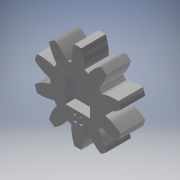
# Autodesk Inventor part: 10_teeth
Saved by Autodesk Inventor 2019 (Build 230136000, 136)
## iProperties
Created: 2020-02-24
Part Number: 10_teeth
Material: Steel
Document SubType Name: Modeling
Designer: Jeff
Categories: <?xml version="1.0" encoding="UTF-16"?> <MemberInstance><Categories><FamilyTemplate><FamilyTemplateParameter ValueType="xs:double" Id="1" ObjectReferenceKey="da_z" ObjectType="kUserParameterObject"/><FamilyTemplateParameter ValueType="xs:double" Id="2" ObjectReferenceKey="da_b" ObjectType="kUserParameterObject"/><FamilyTemplateParameter ValueType="xs:double" Id="3" ObjectReferenceKey="da_beta" ObjectType="kUserParameterObject"/><FamilyTemplateParameter ValueType="xs:double" Id="4" ObjectReferenceKey="da_da" ObjectType="kUserParameterObject"/><FamilyTemplateParameter ValueType="xs:double" Id="5" ObjectReferenceKey="da_aw" ObjectType="kUserParameterObject"/><FamilyTemplateParameter ValueType="xs:string" Id="6" ObjectReferenceKey="EAIAABAAAACIAQAAAAAAAIAAAAAAAAAA" ObjectType="83910656" SubObjectId="SurfaceGeometry"/></FamilyTemplate><ParamToTemplateMap><ParamToTemplate CategoryParameter="//CategoryParameter[@InternalName='046C89C9-8512-4d59-83FE-43B91F4F132A']" TemplateParameter="1"/><ParamToTemplate CategoryParameter="//CategoryParameter[@InternalName='2552DF32-E462-4b46-AEBF-C6C7768E72AC']" TemplateParameter="2"/><ParamToTemplate CategoryParameter="//CategoryParameter[@InternalName='C9EE641D-15FC-4fae-A226-E94C4372FDD7']" TemplateParameter="3"/><ParamToTemplate><ParamToTemplate CategoryParameter="//CategoryParameter[@InternalName='00B6519A-459B-49c7-AD84-2E56D39A5744']" ConstantValue="0.000000"/></ParamToTemplate><ParamToTemplate><ParamToTemplate CategoryParameter="//CategoryParameter[@InternalName='04B31F0E-C7A6-4894-AA32-9629BEFACF47']" ConstantValue="1.000000"/></ParamToTemplate><ParamToTemplate><ParamToTemplate CategoryParameter="//CategoryParameter[@InternalName='43CBEC2E-7847-49e7-A936-2F7889FCB2D9']" ConstantValue="0.250000"/></ParamToTemplate><ParamToTemplate><ParamToTemplate CategoryParameter="//CategoryParameter[@InternalName='B1EFC894-105D-4ebd-86BF-FA20ED196853']" ConstantValue="0.350000"/></ParamToTemplate><ParamToTemplate><ParamToTemplate CategoryParameter="//CategoryParameter[@InternalName='51175063-3D10-4879-93E8-6246FE8B403D']" ConstantValue="2060000000.000000"/></ParamToTemplate><ParamToTemplate><ParamToTemplate CategoryParameter="//CategoryParameter[@InternalName='A3A52E27-4454-46a9-B0BD-C932399B70AF']" ConstantValue="0.300000"/></ParamToTemplate><ParamToTemplate><ParamToTemplate CategoryParameter="//CategoryParameter[@InternalName='91B76062-C214-41d9-B1B9-14D2AB99603D']" ConstantValue="0.300000"/></ParamToTemplate><ParamToTemplate><ParamToTemplate CategoryParameter="//CategoryParameter[@InternalName='374E806E-8B8A-4dda-A9AA-1039D6500AD2']" ConstantValue="3.333333"/></ParamToTemplate><ParamToTemplate><ParamToTemplate CategoryParameter="//CategoryParameter[@InternalName='2D373A89-B862-43d6-8D0B-0CBF12AB9F6C']" ConstantValue="0.349066"/></ParamToTemplate><ParamToTemplate CategoryParameter="//CategoryParameter[@InternalName='37777632-D6A2-4fac-9D53-DB8ACD95C989']" TemplateParameter="4"/><ParamToTemplate CategoryParameter="//CategoryParameter[@InternalName='FD1017F1-B727-4f7e-9707-0F86F1FF9423']" TemplateParameter="5"/><ParamToTemplate><ParamToTemplate CategoryParameter="//CategoryParameter[@InternalName='9E1B4470-B2D3-4ff1-B813-535BB4CDF51A']" ConstantValue="3520000.000000"/></ParamToTemplate><ParamToTemplate><ParamToTemplate CategoryParameter="//CategoryParameter[@InternalName='F8452263-BFF6-458c-9FB1-07C4B99E95CD']" ConstantValue="11400000.000000"/></ParamToTemplate><ParamToTemplate><ParamToTemplate CategoryParameter="//CategoryParameter[@InternalName='3E3BB259-FD49-497f-8171-6EBC954A3479']" ConstantValue="2.000000"/></ParamToTemplate><ParamToTemplate CategoryParameter="//CategoryParameter[@InternalName='27C3BAF2-7550-4e4b-AE2C-0DB134B7D9B7']" TemplateParameter="6"/></ParamToTemplateMap><Category DisplayName="Gear" InternalName="DC85795E-93AB-48d5-8EEE-5A27447B64BD" Mnemonic="Gear"><CategoryParameter DisplayName="z" InternalName="046C89C9-8512-4d59-83FE-43B91F4F132A" Mnemonic="z"/><CategoryParameter DisplayName="b" InternalName="2552DF32-E462-4b46-AEBF-C6C7768E72AC" Mnemonic="b"/><CategoryParameter DisplayName="||b|" InternalName="C9EE641D-15FC-4fae-A226-E94C4372FDD7" Mnemonic="beta"/><CategoryParameter DisplayName="x" InternalName="00B6519A-459B-49c7-AD84-2E56D39A5744" Mnemonic="x"/><CategoryParameter DisplayName="a*" InternalName="04B31F0E-C7A6-4894-AA32-9629BEFACF47" Mnemonic="a"/><CategoryParameter DisplayName="c*" InternalName="43CBEC2E-7847-49e7-A936-2F7889FCB2D9" Mnemonic="c"/><CategoryParameter DisplayName="r|.f|*" InternalName="B1EFC894-105D-4ebd-86BF-FA20ED196853" Mnemonic="rf"/><CategoryParameter DisplayName="E" InternalName="51175063-3D10-4879-93E8-6246FE8B403D" Mnemonic="E"/><CategoryParameter DisplayName="||m|" InternalName="A3A52E27-4454-46a9-B0BD-C932399B70AF" Mnemonic="mi"/><Category DisplayName="SpurGear" InternalName="26C5A22E-A91E-4dfd-A3B3-23CCAFAE1764" Mnemonic="SpurGear"><CategoryParameter DisplayName="m" InternalName="91B76062-C214-41d9-B1B9-14D2AB99603D" Mnemonic="m"/><CategoryParameter DisplayName="P" InternalName="374E806E-8B8A-4dda-A9AA-1039D6500AD2" Mnemonic="PP"/><CategoryParameter DisplayName="||a|" InternalName="2D373A89-B862-43d6-8D0B-0CBF12AB9F6C" Mnemonic="alpha"/><CategoryParameter DisplayName="d|.a|" InternalName="37777632-D6A2-4fac-9D53-DB8ACD95C989" Mnemonic="da"/><CategoryParameter DisplayName="a|.w|" InternalName="FD1017F1-B727-4f7e-9707-0F86F1FF9423" Mnemonic="aw"/><CategoryParameter DisplayName="||s||.Flim|" InternalName="9E1B4470-B2D3-4ff1-B813-535BB4CDF51A" Mnemonic="sFlim"/><CategoryParameter DisplayName="||s||.Hlim|" InternalName="F8452263-BFF6-458c-9FB1-07C4B99E95CD" Mnemonic="sHlim"/><CategoryParameter DisplayName="type" InternalName="3E3BB259-FD49-497f-8171-6EBC954A3479" Mnemonic="type"/><CategoryParameter DisplayName="PitchDiameter" InternalName="27C3BAF2-7550-4e4b-AE2C-0DB134B7D9B7" Mnemonic="IDS_PITCHDIAM"/></Category></Category></Categories></MemberInstance>
Density: 1 g/cm^3
Appearance: Steel
Author: Jeff
Autodesk Inventor part; units mm, degrees
sketch "Sketch1" plane through (0, 0, 0) normal (0, 0, 1) x (1, 0, 0)
  circle A0 centre (0, 0) radius 18
  dimension "d0" = 36
  constraints: 1 centre point
  measures "d0" diameter of A0
extrude "Extrusion1" add sketch "Sketch1" along normal blind 10
ref_plane "Work Plane2" through (0, 0, 5) normal (0, 0, 1) x (1, 0, 0)
sketch "Sketch2" plane through (0, 0, 0) normal (0, 0, -1) x (-1, 0, 0)
  circle A0 centre (0, 0) radius 18 projected
  circle A1 centre (0, 0) radius 15
  dimension "d3" = 30
  constraints: 1 centre point, 1 coincident
  measures "d3" diameter of A1
surface extrude "Pitch Diameter" sketch "Sketch2" against normal through all shown no curves A1
ref_plane "Work Plane8" through (0, 0, 0) normal (0.9510565, 0.309017, 0) x (0, 0, 1)
ref_plane "Work Plane9" through (0, 0, 0) normal (1, 0, 0) x (0, 1, 0)
spur gear teeth "Spur Gear" teeth 10 pitch diameter 30 tip diameter 36 root diameter 22.5 face width 10 start plane through (0, 0, 0) normal (0, 0, -1) x (-1, 0, 0)
sketch "Sketch3" plane through (0, 0, 10) normal (0, 0, 1) x (1, 0, 0)
  line L0 (-5, 5) -> (5, 5)
  line L1 (5, 5) -> (5, -5)
  line L2 (5, -5) -> (-5, -5)
  line L3 (-5, -5) -> (-5, 5)
  line L4 (-5, -2.9696) -> (5, -2.9696) construction
  line L5 (5, -2.9696) -> (5, -12.9696) construction
  line L6 (5, -12.9696) -> (-5, -12.9696) construction
  line L7 (-5, -12.9696) -> (-5, -2.9696) construction
  arc A0 (-2.6263, -10.9392) -> (-1.4123, -17.9445) centre (13.7859, -11.7029) ccw projected
  line L8 (-2.6263, -10.9392) -> (-2.6263, -5)
  line L9 (-0.3331, -9.4684) -> (-1.7966, -9.4684)
  line L10 (-1.7966, -9.4684) -> (-1.7966, -9.162)
  line L11 (-1.7966, -9.162) -> (-1.252, -9.162)
  line L12 (-1.252, -9.162) -> (-1.252, -7.1515)
  line L13 (-1.252, -7.1515) -> (-1.7966, -7.1515)
  line L14 (-1.7966, -7.1515) -> (-1.7966, -6.8768)
  spline S0 degree 2 poles (-1.7966, -6.8768) (-1.4878, -6.8768) (-1.1961, -6.7018) (-1.1767, -6.4586) knots 0 0 0 1 2 2 2
  line L15 (-1.1767, -6.4586) -> (-0.8655, -6.4586)
  line L16 (-0.8655, -6.4586) -> (-0.8655, -9.162)
  line L17 (-0.8655, -9.162) -> (-0.3331, -9.162)
  line L18 (-0.3331, -9.162) -> (-0.3331, -9.4684)
  spline S1 degree 2 poles (2.0859, -7.9684) (2.0859, -8.7755) (1.6167, -9.5316) (1.128, -9.5316) knots 0 0 0 1 2 2 2
  spline S2 degree 2 poles (1.128, -9.5316) (0.6321, -9.5316) (0.1677, -8.7609) (0.1677, -7.9708) knots 0 0 0 1 2 2 2
  spline S3 degree 2 poles (0.1677, -7.9708) (0.1677, -7.1588) (0.637, -6.4076) (1.128, -6.4076) knots 0 0 0 1 2 2 2
  spline S4 degree 2 poles (1.128, -6.4076) (1.6216, -6.4076) (2.0859, -7.1855) (2.0859, -7.9684) knots 0 0 0 1 2 2 2
  spline S5 degree 2 poles (1.5705, -8.8825) (1.6288, -8.7342) (1.6775, -8.2771) (1.6775, -7.9684) knots 0 0 0 1 2 2 2
  spline S6 degree 2 poles (1.6775, -7.9684) (1.6775, -7.6596) (1.6288, -7.205) (1.5681, -7.0518) knots 0 0 0 1 2 2 2
  spline S7 degree 2 poles (1.5681, -7.0518) (1.5073, -6.8987) (1.2958, -6.7407) (1.128, -6.7407) knots 0 0 0 1 2 2 2
  spline S8 degree 2 poles (1.128, -6.7407) (0.9603, -6.7407) (0.7439, -6.8987) (0.6807, -7.0567) knots 0 0 0 1 2 2 2
  spline S9 degree 2 poles (0.6807, -7.0567) (0.6199, -7.2099) (0.5762, -7.6766) (0.5762, -7.9708) knots 0 0 0 1 2 2 2
  spline S10 degree 2 poles (0.5762, -7.9708) (0.5762, -8.2868) (0.6151, -8.7099) (0.6783, -8.8752) knots 0 0 0 1 2 2 2
  spline S11 degree 2 poles (0.6783, -8.8752) (0.7366, -9.0308) (0.953, -9.1985) (1.128, -9.1985) knots 0 0 0 1 2 2 2
  spline S12 degree 2 poles (1.128, -9.1985) (1.2934, -9.1985) (1.5097, -9.0405) (1.5705, -8.8825) knots 0 0 0 1 2 2 2
  point P0 (0, 0)
  point P1 (0, 5)
  point P2 (5, 0)
  point P3 (-2.6263, -7.9696)
  point P4 (0, -2.9696)
  point P5 (-5, -7.9696)
  dimension "d49" = 10
  dimension "d50" = 10
  dimension "d57" = 10
  dimension "d58" = 10
  constraints: 10 end point, 5 midpoint, 2 horizontal, 2 horizontal alignment, 2 parallel, 2 perpendicular, 2 vertical alignment, 1 point on line, 2 other
  measures "d49" distance of L1.end L2.end
  measures "d50" distance of L0.end L1.end
  measures "d57" distance between parallel lines of L5 L7
  measures "d58" distance between parallel lines of L4 L6
extrude "Extrusion2" cut sketch "Sketch3" against normal blind 4
sketch "Sketch4" plane through (0, 0, 0) normal (0, 0, -1) x (-1, 0, 0)
  circle A0 centre (0, 0) radius 7.5
  dimension "d53" = 15
  constraints: 1 centre point, 1 coincident
  measures "d53" diameter of A0
extrude "Extrusion3" cut sketch "Sketch4" against normal blind 4
equation "\"d0\" = da_da"
equation "\"d1\" = da_b"
equation "\"d3\" = da_dw"
equation "\"da_da\" = 36"
equation "\"da_b\" = 10"
equation "\"da_dw\" = 30"
body "Solid1"
body "Srf1"
